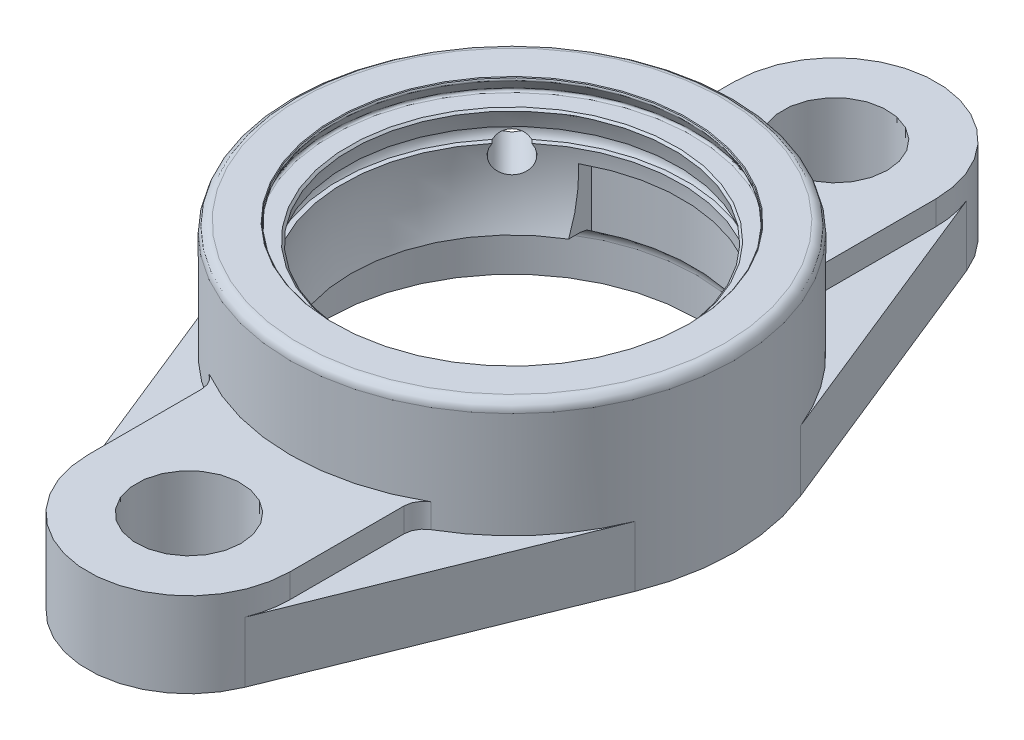
# Autodesk Inventor part: FL 205/Y++35.7_h
Saved by Autodesk Inventor 2019 (Build 230136000, 136)
## iProperties
Created: 2024-04-15
Part Number: FL 205/Y++35.7_h
Material: Generic
Catalog Web Link: www.cadenas.de
Description: AFC_011-012_AFV_011_AFP_011 h-Oval flanged housings for Y-bearings
Vendor: SKF
Document SubType Name: Modeling
Designer: psAdmin
Manufacturer: SKF
Mass: 60.0993 g
Surface Area: 206.448 cm^2
Volume: 60.0993 cm^3
Density: 1 g/cm^3
Appearance: PSOLRGB-175-175-175
Category: PARTsolutions
Company: SKF
Title: FL 205/Y++35.7_h
Author: Cadenas PARTsolutions
Comments: Oval flanged housings for Y-bearings
PSOL_IDENT_0: {$CADENAS_DATA/23d-libs/skf/bearings_units_and_housings/bearing_units/ball_bearing_units/y-units/y-b
PSOL_IDENT_1: earing_oval_flanged_units_parts/ayf_002hc_hh_hy_ayd_001hp_housing.prj},205 {VTYP=3D},{NB=FL 205/Y++3
PSOL_IDENT_2: 5.7_h},{LINA=FL 205/Y++35.7_h},{NN=AFC_011-012_AFV_011_AFP_011 h},{DATE=10.03.2023 09:37:08},{GEOMDA
PSOL_IDENT_3: TE=02.03.2023 09:48:21},{VERSION=},{LINEID=6030},{WBVAR=COVER,T},{WBNUMERIC=T}  {NB=FL 205/Y++35.7_h
PSOL_IDENT_4: },{LINA=FL 205/Y++35.7_h},{KT=DUMMY},{DESIGNATION=FL 205/Y},{COVER=},{DAAX=0.000},{T=35.700},{SS1=19
PSOL_IDENT_5: .700},{D=52.000},{DA=0.000},{DB=0.000},{DB1=68.000},{DB2=0.000},{A=27.000},{A1=13.000},{A2=0.000},{A
PSOL_IDENT_6: 3=0.000},{A5=20.500},{J=99.000},{H=130.000},{L=68.000},{N=16.000},{RG=1/4-28 UNF},{R1=17.500},{DN=6.
PSOL_IDENT_7: 6},{RA=45.000},{SWN=7.940},{GN=1/4-28 UNF},{J6=0.000},{J7=0.000},{N1=0.000},{N4=0.000},{MASS=0.610},
PSOL_IDENT_8: {G=14.000},{GIN=0.563},{EC=ECY 205},{AEC=23.000},{DEC=49.100},{D1EC=54.000},{D2EC=55.500},{DESIGN=uc
PSOL_IDENT_9: fl/ukfl_205},{ECPN=},{SUPPRESSED=unsuppressed},{R2=0.000},{H1=0.000},{L1=0.000},{H2=0.000},{R3=0.000
PSOL_IDENT_10: },{H3=0.000},{L2=0.000},{H4=0.000},{H5=0.000},{H6=0.000},{R4=0.000},{L3=0.000},{H7=0.000},{H8=0.000}
PSOL_IDENT_11: ,{H9=0.000},{L4=0.000},{H10=0.000},{H11=0.000},{H12=0.000},{DC=0.000},{DD=0.000},{R5=0.000},{R6=0.00
PSOL_IDENT_12: 0},{X=0.000},{Y=0.000},{R7=0.000},{X2=0.000},{Y2=0.000},{E=0.000},{TALG=35.7,35.8}
NB: FL 205/Y++35.7_h
NN: AFC_011-012_AFV_011_AFP_011 h
NT: Oval flanged housings for Y-bearings
NBSYN: $DESIGNATION.+$COVER.+$T._h
LINA: FL 205/Y++35.7_h
CATALOG: SKF
DESIGNATION: FL 205/Y
COVER: No End Cover
DAAX: 0
T: 35.7
D: 52
DA: 0
DB: 0
DB1: 68
DB2: 0
A: 27
A1: 13
A2: 0
A3: 0
A5: 20.5
J: 99
H: 130
L: 68
N: 16
RG: 1/4-28 UNF
R1: 17.5
DN: 6.6
RA: 45
SWN: 7.94
GN: 1/4-28 UNF
J6: 0
J7: 0
N1: 0
N4: 0
MASS: 0.61
G: 14
GIN: 0.563
EC: ECY 205
AEC: 23
DEC: 49.1
D1EC: 54
D2EC: 55.5
R2: 0
H1: 0
L1: 0
H2: 0
R3: 0
H3: 0
L2: 0
H4: 0
H5: 0
H6: 0
R4: 0
L3: 0
H7: 0
H8: 0
H9: 0
L4: 0
H10: 0
H11: 0
H12: 0
DC: 0
DD: 0
R5: 0
R6: 0
X: 0
Y: 0
R7: 0
X2: 0
Y2: 0
E: 0
SUPPLIER: SKF
ARTICLENO: FL 205/Y++35.7_h
BOMINFO: FL 205/Y++35.7_h
CREATOR: CADENAS GmbH
Autodesk Inventor part; units mm, degrees
sketch "Sketch_1" plane through (0, 0, 0) normal (0, 0, 1) x (1, 0, 0)
  line L0 (0, 0) -> (0, 27)
  line L1 (0, 27) -> (32.5, 27)
  arc A0 (34, 25.5) -> (32.5, 27) centre (32.5, 25.5) ccw
  line L2 (34, 25.5) -> (34, 0)
  line L3 (34, 0) -> (0, 0)
  line L4 (0, 0) -> (0, 27)
  constraints: 10 end point, 2 point on circle, 1 centre point
revolve "Revolution1" add sketch "Sketch_1" angle 360 about axis through (0, 0, 0) along (0, -1, 0)
sketch "Sketch_2" plane through (0, 0, 0) normal (0, 1, 0) x (-1, 0, 0)
  arc A0 (31.5362, -12.7071) -> (31.5362, 12.7071) centre (0, 0) ccw
  line L0 (31.5362, 12.7071) -> (14.3768, 55.2929)
  arc A1 (14.3768, 55.2929) -> (-14.3768, 55.2929) centre (0, 49.5) ccw
  line L1 (-14.3768, 55.2929) -> (-31.5362, 12.7071)
  arc A2 (-31.5362, 12.7071) -> (-31.5362, -12.7071) centre (0, 0) ccw
  line L2 (-31.5362, -12.7071) -> (-14.3768, -55.2929)
  arc A3 (-14.3768, -55.2929) -> (14.3768, -55.2929) centre (0, -49.5) ccw
  line L3 (14.3768, -55.2929) -> (31.5362, -12.7071)
  constraints: 8 end point, 8 point on circle, 4 centre point
extrude "Extrusion1" add sketch "Sketch_2" along normal blind 9.3
sketch "Sketch_3" plane through (0, 0, 0) normal (0, 1, 0) x (-1, 0, 0)
  arc A0 (17, -29.4449) -> (17, 29.4449) centre (0, 0) ccw
  arc A1 (15.5, 32.0429) -> (17, 29.4449) centre (18.5, 32.0429) ccw
  line L0 (15.5, 32.0429) -> (15.5, 49.5)
  arc A2 (15.5, 49.5) -> (-15.5, 49.5) centre (0, 49.5) ccw
  line L1 (-15.5, 49.5) -> (-15.5, 32.0429)
  arc A3 (-17, 29.4449) -> (-15.5, 32.0429) centre (-18.5, 32.0429) ccw
  arc A4 (-17, 29.4449) -> (-17, -29.4449) centre (0, 0) ccw
  arc A5 (-15.5, -32.0429) -> (-17, -29.4449) centre (-18.5, -32.0429) ccw
  line L2 (-15.5, -32.0429) -> (-15.5, -49.5)
  arc A6 (-15.5, -49.5) -> (15.5, -49.5) centre (0, -49.5) ccw
  line L3 (15.5, -49.5) -> (15.5, -32.0429)
  arc A7 (17, -29.4449) -> (15.5, -32.0429) centre (18.5, -32.0429) ccw
  constraints: 16 point on circle, 8 centre point, 8 end point
extrude "Extrusion2" add sketch "Sketch_3" along normal blind 13
sketch "Sketch4" plane through (0, 0, 49.5) normal (0, -1, 0) x (1, 0, 0)
  point P0 (0, 0)
hole "Hole1" at (0, 0, 49.5) direction (0, 1, 0) diameter 16 depth 13
sketch "Sketch5" plane through (0, 0, 49.5) normal (0, -1, 0) x (1, 0, 0)
  point P0 (0, -99)
hole "Hole2" at (0, 0, -49.5) direction (0, 1, 0) diameter 16 depth 13
sketch "Sketch_6" plane through (0, 0, 0) normal (0, 0, 1) x (1, 0, 0)
  line L0 (0, 0) -> (0, 27)
  line L1 (0, 27) -> (27.19, 27)
  line L2 (27.19, 27) -> (27.0893, 26.8993)
  arc A0 (27.0893, 26.8993) -> (27.0416, 26.5372) centre (27.3014, 26.6872) ccw
  line L3 (27.0416, 26.5372) -> (27.958, 24.95)
  arc A1 (27.6982, 24.5) -> (27.958, 24.95) centre (27.6982, 24.8) ccw
  line L4 (27.6982, 24.5) -> (24.9997, 24.5)
  line L5 (24.9997, 24.5) -> (24.6797, 24.18)
  arc A2 (25.3787, 21.65) -> (24.6797, 24.18) centre (0, 16) ccw
  line L6 (25.3787, 21.65) -> (26.5612, 21.65)
  arc A3 (26.5612, 19.15) -> (26.5612, 21.65) centre (25, 20.4) ccw
  line L7 (26.5612, 19.15) -> (25.8085, 19.15)
  arc A4 (24.6564, 7.75) -> (25.8085, 19.15) centre (0, 16) ccw
  line L8 (24.6564, 7.75) -> (26.25, 7.75)
  arc A5 (28.25, 5.75) -> (26.25, 7.75) centre (26.25, 5.75) ccw
  line L9 (28.25, 5.75) -> (28.25, 0)
  line L10 (28.25, 0) -> (0, 0)
  line L11 (0, 0) -> (0, 27)
  constraints: 24 end point, 12 point on circle, 6 centre point
revolve "Revolution2" cut sketch "Sketch_6" angle 360 about axis through (0, 0, 0) along (0, -1, 0)
sketch "Sketch_7" plane through (0, 0, 0) normal (0, 1, 0) x (-1, 0, 0)
  line L0 (12.545, -24.7525) -> (12.545, 24.7525)
  arc A0 (12.545, 24.7525) -> (-12.545, 24.7525) centre (0, 0) ccw
  line L1 (-12.545, 24.7525) -> (-12.545, -24.7525)
  arc A1 (-12.545, -24.7525) -> (12.545, -24.7525) centre (0, 0) ccw
  constraints: 4 end point, 4 point on circle, 2 centre point
extrude "Extrusion3" cut sketch "Sketch_7" along normal blind 17
sketch "Sketch_8" plane through (0, 0, 0) normal (0.7071, 0, -0.7071) x (-0.7071, 0, -0.7071)
  line L0 (34, 17.5) -> (0, 17.5)
  line L1 (0, 17.5) -> (0, 20.205)
  line L2 (0, 20.205) -> (34, 20.205)
  line L3 (34, 20.205) -> (34, 17.5)
  line L4 (34, 17.5) -> (0, 17.5)
  constraints: 10 end point
revolve "Revolution3" cut sketch "Sketch_8" angle 360 about axis through (-24.0416, 17.5, -24.0416) along (-0.7071, 0, -0.7071)
sketch "Sketch_9" plane through (-27.2, 0, 0) normal (1, 0, 0) x (0, 0, -1)
  arc A0 (-13.5973, 18.0793) -> (-13.5037, 17.9857) centre (-13.5037, 18.0793) ccw
  line L0 (-13.5037, 17.9857) -> (-12.3597, 17.9857)
  arc A1 (-12.3597, 17.9857) -> (-12.2661, 18.0793) centre (-12.3597, 18.0793) ccw
  line L1 (-12.2661, 18.0793) -> (-12.2661, 18.635)
  arc A2 (-12.1725, 18.7286) -> (-12.2661, 18.635) centre (-12.1725, 18.635) ccw
  line L2 (-12.1725, 18.7286) -> (-8.0511, 18.7286)
  arc A3 (-7.9575, 18.635) -> (-8.0511, 18.7286) centre (-8.0511, 18.635) ccw
  line L3 (-7.9575, 18.635) -> (-7.9575, 17.4078)
  arc A4 (-8.1224, 17.2429) -> (-7.9575, 17.4078) centre (-8.1224, 17.4078) ccw
  line L4 (-8.1224, 17.2429) -> (-9.2783, 17.2429)
  arc A5 (-9.4432, 17.4078) -> (-9.2783, 17.2429) centre (-9.2783, 17.4078) ccw
  line L5 (-9.4432, 17.4078) -> (-9.4432, 17.4486)
  arc A6 (-9.4432, 17.4486) -> (-9.6081, 17.6135) centre (-9.6081, 17.4486) ccw
  line L6 (-9.6081, 17.6135) -> (-10.764, 17.6135)
  arc A7 (-10.764, 17.6135) -> (-10.9289, 17.4486) centre (-10.764, 17.4486) ccw
  line L7 (-10.9289, 17.4486) -> (-10.9289, 16.2927)
  arc A8 (-10.9289, 16.2927) -> (-10.764, 16.1278) centre (-10.764, 16.2927) ccw
  line L8 (-10.764, 16.1278) -> (-9.6081, 16.1278)
  arc A9 (-9.6081, 16.1278) -> (-9.4432, 16.2927) centre (-9.6081, 16.2927) ccw
  line L9 (-9.4432, 16.2927) -> (-9.4432, 16.3351)
  arc A10 (-9.2783, 16.5) -> (-9.4432, 16.3351) centre (-9.2783, 16.3351) ccw
  line L10 (-9.2783, 16.5) -> (-8.1224, 16.5)
  arc A11 (-7.9575, 16.3351) -> (-8.1224, 16.5) centre (-8.1224, 16.3351) ccw
  line L11 (-7.9575, 16.3351) -> (-7.9575, 15.8507)
  arc A12 (-8.0511, 15.7571) -> (-7.9575, 15.8507) centre (-8.0511, 15.8507) ccw
  line L12 (-8.0511, 15.7571) -> (-8.5354, 15.7571)
  arc A13 (-8.5354, 15.7571) -> (-8.7003, 15.5922) centre (-8.5354, 15.5922) ccw
  line L13 (-8.7003, 15.5922) -> (-8.7003, 13.6222)
  arc A14 (-8.7003, 13.6222) -> (-8.6067, 13.5286) centre (-8.6067, 13.6222) ccw
  line L14 (-8.6067, 13.5286) -> (-5.9674, 13.5286)
  arc A15 (-5.9674, 13.5286) -> (-5.8025, 13.6935) centre (-5.9674, 13.6935) ccw
  line L15 (-5.8025, 13.6935) -> (-5.8025, 14.3673)
  line L16 (-5.8025, 14.3673) -> (-4.9667, 14.3673)
  line L17 (-4.9667, 14.3673) -> (-4.9667, 13.8331)
  arc A16 (-4.9667, 13.8331) -> (-4.6622, 13.5286) centre (-4.6622, 13.8331) ccw
  line L18 (-4.6622, 13.5286) -> (-1.883, 13.5286)
  arc A17 (-1.883, 13.5286) -> (-1.6677, 13.6178) centre (-1.883, 13.8331) ccw
  line L19 (-1.6677, 13.6178) -> (0.7541, 16.0395)
  arc A18 (1.274, 15.8241) -> (0.7541, 16.0395) centre (0.9694, 15.8241) ccw
  line L20 (1.274, 15.8241) -> (1.274, 13.8331)
  arc A19 (1.274, 13.8331) -> (1.5786, 13.5286) centre (1.5786, 13.8331) ccw
  line L21 (1.5786, 13.5286) -> (4.0887, 13.5286)
  arc A20 (4.0887, 13.5286) -> (4.3933, 13.8331) centre (4.0887, 13.8331) ccw
  line L22 (4.3933, 13.8331) -> (4.3933, 14.3673)
  line L23 (4.3933, 14.3673) -> (5.229, 14.3673)
  line L24 (5.229, 14.3673) -> (5.229, 13.6244)
  arc A21 (5.229, 13.6244) -> (5.3248, 13.5286) centre (5.3248, 13.6244) ccw
  line L25 (5.3248, 13.5286) -> (12.9331, 13.5286)
  arc A22 (12.9331, 13.5286) -> (13.029, 13.6244) centre (12.9331, 13.6244) ccw
  line L26 (13.029, 13.6244) -> (13.029, 15.6613)
  arc A23 (13.029, 15.6613) -> (12.9331, 15.7571) centre (12.9331, 15.6613) ccw
  line L27 (12.9331, 15.7571) -> (10.8962, 15.7571)
  arc A24 (10.8962, 15.7571) -> (10.8004, 15.6613) centre (10.8962, 15.6613) ccw
  line L28 (10.8004, 15.6613) -> (10.8004, 14.3673)
  arc A25 (10.7046, 14.2714) -> (10.8004, 14.3673) centre (10.7046, 14.3673) ccw
  line L29 (10.7046, 14.2714) -> (7.9248, 14.2714)
  arc A26 (7.829, 14.3673) -> (7.9248, 14.2714) centre (7.9248, 14.3673) ccw
  line L30 (7.829, 14.3673) -> (7.829, 16.4042)
  arc A27 (7.9248, 16.5) -> (7.829, 16.4042) centre (7.9248, 16.4042) ccw
  line L31 (7.9248, 16.5) -> (12.1903, 16.5)
  arc A28 (12.1903, 16.5) -> (12.2861, 16.5958) centre (12.1903, 16.5958) ccw
  line L32 (12.2861, 16.5958) -> (12.2861, 19.3756)
  arc A29 (12.2861, 19.3756) -> (12.1903, 19.4714) centre (12.1903, 19.3756) ccw
  line L33 (12.1903, 19.4714) -> (6.4391, 19.4714)
  arc A30 (6.4391, 19.4714) -> (6.3433, 19.3756) centre (6.4391, 19.3756) ccw
  line L34 (6.3433, 19.3756) -> (6.3433, 18.0793)
  arc A31 (6.3433, 18.0793) -> (6.4369, 17.9857) centre (6.4369, 18.0793) ccw
  line L35 (6.4369, 17.9857) -> (9.2189, 17.9857)
  arc A32 (9.2189, 17.9857) -> (9.3147, 18.0815) centre (9.2189, 18.0815) ccw
  line L36 (9.3147, 18.0815) -> (9.3147, 18.6327)
  arc A33 (9.4105, 18.7286) -> (9.3147, 18.6327) centre (9.4105, 18.6327) ccw
  line L37 (9.4105, 18.7286) -> (9.9617, 18.7286)
  arc A34 (10.0575, 18.6327) -> (9.9617, 18.7286) centre (9.9617, 18.6327) ccw
  line L38 (10.0575, 18.6327) -> (10.0575, 17.3387)
  arc A35 (9.9617, 17.2429) -> (10.0575, 17.3387) centre (9.9617, 17.3387) ccw
  line L39 (9.9617, 17.2429) -> (5.3226, 17.2429)
  arc A36 (5.3226, 17.2429) -> (5.229, 17.1493) centre (5.3226, 17.1493) ccw
  line L40 (5.229, 17.1493) -> (5.229, 14.6072)
  line L41 (5.229, 14.6072) -> (4.3933, 14.6072)
  line L42 (4.3933, 14.6072) -> (4.3933, 15.5751)
  arc A37 (4.3933, 15.5751) -> (4.2113, 15.7571) centre (4.2113, 15.5751) ccw
  line L43 (4.2113, 15.7571) -> (3.9475, 15.7571)
  line L44 (3.9475, 15.7571) -> (3.9475, 17.2429)
  line L45 (3.9475, 17.2429) -> (4.2113, 17.2429)
  arc A38 (4.2113, 17.2429) -> (4.3933, 17.4249) centre (4.2113, 17.4249) ccw
  line L46 (4.3933, 17.4249) -> (4.3933, 19.1669)
  arc A39 (4.3933, 19.1669) -> (4.0887, 19.4714) centre (4.0887, 19.1669) ccw
  line L47 (4.0887, 19.4714) -> (1.5786, 19.4714)
  arc A40 (1.5786, 19.4714) -> (1.274, 19.1669) centre (1.5786, 19.1669) ccw
  line L48 (1.274, 19.1669) -> (1.274, 16.9758)
  arc A41 (0.9633, 16.8471) -> (1.274, 16.9758) centre (1.092, 16.9758) ccw
  line L49 (0.9633, 16.8471) -> (-1.5039, 19.3143)
  arc A42 (-1.5039, 19.3143) -> (-1.8832, 19.4714) centre (-1.8832, 18.9351) ccw
  line L50 (-1.8832, 19.4714) -> (-3.9193, 19.4714)
  arc A43 (-3.9193, 19.4714) -> (-4.2239, 19.1669) centre (-3.9193, 19.1669) ccw
  line L51 (-4.2239, 19.1669) -> (-4.2239, 18.2903)
  arc A44 (-4.2239, 18.2903) -> (-3.9193, 17.9857) centre (-3.9193, 18.2903) ccw
  line L52 (-3.9193, 17.9857) -> (-1.883, 17.9857)
  arc A45 (-1.6677, 17.8965) -> (-1.883, 17.9857) centre (-1.883, 17.6811) ccw
  line L53 (-1.6677, 17.8965) -> (-1.2706, 17.4995)
  arc A46 (-1.2706, 17.0687) -> (-1.2706, 17.4995) centre (-1.486, 17.2841) ccw
  line L54 (-1.2706, 17.0687) -> (-2.4251, 15.9142)
  arc A47 (-2.8043, 15.7571) -> (-2.4251, 15.9142) centre (-2.8043, 16.2935) ccw
  line L55 (-2.8043, 15.7571) -> (-4.6622, 15.7571)
  arc A48 (-4.6622, 15.7571) -> (-4.9667, 15.4526) centre (-4.6622, 15.4526) ccw
  line L56 (-4.9667, 15.4526) -> (-4.9667, 14.6072)
  line L57 (-4.9667, 14.6072) -> (-5.8025, 14.6072)
  line L58 (-5.8025, 14.6072) -> (-5.8025, 15.5922)
  arc A49 (-5.8025, 15.5922) -> (-5.9674, 15.7571) centre (-5.9674, 15.5922) ccw
  line L59 (-5.9674, 15.7571) -> (-6.0097, 15.7571)
  arc A50 (-6.1746, 15.9221) -> (-6.0097, 15.7571) centre (-6.0097, 15.9221) ccw
  line L60 (-6.1746, 15.9221) -> (-6.1746, 17.0779)
  arc A51 (-6.0097, 17.2429) -> (-6.1746, 17.0779) centre (-6.0097, 17.0779) ccw
  line L61 (-6.0097, 17.2429) -> (-5.9674, 17.2429)
  arc A52 (-5.9674, 17.2429) -> (-5.8025, 17.4078) centre (-5.9674, 17.4078) ccw
  line L62 (-5.8025, 17.4078) -> (-5.8025, 19.3778)
  arc A53 (-5.8025, 19.3778) -> (-5.8961, 19.4714) centre (-5.8961, 19.3778) ccw
  line L63 (-5.8961, 19.4714) -> (-13.5037, 19.4714)
  arc A54 (-13.5037, 19.4714) -> (-13.5973, 19.3778) centre (-13.5037, 19.3778) ccw
  line L64 (-13.5973, 19.3778) -> (-13.5973, 18.0793)
  constraints: 130 end point, 110 point on circle, 55 centre point
extrude "Extrusion4" add sketch "Sketch_9" against normal blind 7
sketch "Sketch_10" plane through (0, 0, 0) normal (0, 0, 1) x (1, 0, 0)
  line L0 (0, 27) -> (0, 0)
  line L1 (-52, 9) -> (-34.2, 9)
  line L2 (-34.2, 9) -> (-34.2, 27)
  line L3 (-34.2, 27) -> (-52, 27)
  line L4 (-52, 27) -> (-52, 9)
  constraints: 10 end point
revolve "Revolution4" cut sketch "Sketch_10" angle 54.4 mid plane about axis through (0, 27, 0) along (0, -1, 0)
ref_plane "brg_XY" through (0, 16, 0) normal (0, 1, 0) x (1, 0, 0)
ref_plane "brg_YZ" through (0, 16, 0) normal (1, 0, 0) x (0, 0, -1)
ref_plane "brg_ZX" through (0, 16, 0) normal (0, 0, -1) x (0, 1, 0)
ref_plane "cover_XY" through (0, 47.5, 0) normal (0, 1, 0) x (1, 0, 0)
ref_plane "cover_YZ" through (0, 47.5, 0) normal (1, 0, 0) x (0, 0, -1)
ref_plane "cover_ZX" through (0, 47.5, 0) normal (0, 0, -1) x (0, 1, 0)
ref_plane "gn_XY" through (-24.0416, 17.5, -24.0416) normal (0.7071, 0, -0.7071) x (-0.7071, 0, -0.7071)
ref_plane "gn_YZ" through (-24.0416, 17.5, -24.0416) normal (-0.7071, 0, -0.7071) x (0, 1, 0)
ref_plane "gn_ZX" through (-24.0416, 17.5, -24.0416) normal (0, 1, 0) x (0.7071, 0, -0.7071)
ref_plane "housing_XY" through (0, 0, 0) normal (0, 1, 0) x (1, 0, 0)
ref_plane "housing_YZ" through (0, 0, 0) normal (1, 0, 0) x (0, 0, -1)
ref_plane "housing_ZX" through (0, 0, 0) normal (0, 0, -1) x (0, 1, 0)
body "Solid1"
